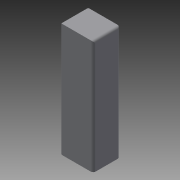
# Autodesk Inventor part: bateria
Saved by Autodesk Inventor 2015 (Build 190159000, 159)
## iProperties
Created: 2015-06-13
Part Number: bateria
Material: Generic
Document SubType Name: Modeling
Designer: Jufo
Density: 1 g/cm^3
Appearance: Default
Author: Jufo
Autodesk Inventor part; units mm, degrees
ref_plane "YZ Plane" through (0, 0, 0) normal (1, 0, 0) x (0, 1, 0)
ref_plane "XZ Plane" through (0, 0, 0) normal (0, 1, 0) x (-1, 0, 0)
ref_plane "XY Plane" through (0, 0, 0) normal (0, 0, 1) x (1, 0, 0)
sketch "Sketch1" plane through (0, 0, 0) normal (0, 1, 0) x (-1, 0, 0)
  line L0 (-13.0395, 8.2682) -> (15.3605, 8.2682)
  line L1 (15.3605, 8.2682) -> (15.3605, -88.7318)
  line L2 (15.3605, -88.7318) -> (-13.0395, -88.7318)
  line L3 (-13.0395, -88.7318) -> (-13.0395, 8.2682)
  point P0 (0, 0)
  dimension "d0" = 28.4
  dimension "d1" = 97
  constraints: 8 end point, 2 perpendicular, 1 horizontal, 1 parallel
  measures "d0" distance of L0.start L0.end
  measures "d1" distance of L0.end L1.end
extrude "Extrusion1" add sketch "Sketch1" along normal blind 23
fillet "Fillet1" radius 2 6 edges at (13.0395, 23, -40.2318) (13.0395, 0, -40.2318) (-15.3605, 23, -40.2318) (-15.3605, 0, -40.2318) (13.0395, 11.5, 8.2682) (-15.3605, 11.5, 8.2682)
body "Solid1"
